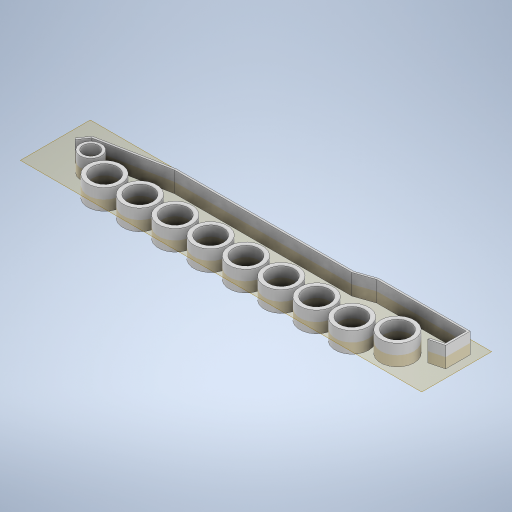
# Autodesk Inventor part: Track_mass_and_inertia
Saved by Autodesk Inventor 2024 (Build 280153000, 153)
## iProperties
Created: 2026-05-25
Part Number: Track_mass_and_inertia
Material: Generic
Document SubType Name: Modeling
Designer: warny
Density: 1 g/cm^3
Appearance: Default
Author: warny
Autodesk Inventor part; units mm, degrees
ref_plane "YZ Plane" through (0, 0, 0) normal (1, 0, 0) x (0, 1, 0)
ref_plane "XY Plane" through (0, 0, 0) normal (0, 0, 1) x (1, 0, 0)
sketch "Sketch1" plane through (0, 0, 0) normal (0, 1, 0) x (-1, 0, 0)
  line L0 (0, -144.8636) -> (0, 84.5516) construction
  line L1 (624.86, 0) -> (-675.46, 0) construction
  line L2 (338.2, 51.778) -> (439.1, -35.05)
  line L3 (439.1, -35.05) -> (421.2, -60.89)
  line L4 (421.2, -60.89) -> (242.5, -95.89)
  line L5 (242.5, -95.89) -> (-209.7, -95.89)
  line L6 (-209.7, -95.89) -> (-256.7, -112.09)
  line L7 (-256.7, -112.09) -> (-489.7, -112.09)
  line L8 (-489.7, -112.09) -> (-489.7, -49.69)
  line L9 (-489.7, -49.69) -> (-453.7, -40.3)
  line L10 (-453.7, -40.3) -> (-431.7, 3.13)
  line L11 (-431.7, 3.13) -> (-349.7, 51.778)
  line L12 (-349.7, 51.778) -> (338.2, 51.778)
  circle A0 centre (393.1, -28.9) radius 27.035
  circle A1 centre (322.2, 6.91) radius 42.8135
  circle A2 centre (232.2, 6.91) radius 42.8135
  circle A3 centre (142.2, 6.91) radius 42.8135
  circle A4 centre (52.2, 6.91) radius 42.8135
  circle A5 centre (-37.8, 6.91) radius 42.8135
  circle A6 centre (-127.8, 6.91) radius 42.8135
  circle A7 centre (-217.8, 6.91) radius 42.8135
  circle A8 centre (-307.8, 6.91) radius 42.8135
  circle A9 centre (-393.7, -22.87) radius 42.8135
  line L13 (435.2892, -31.7707) -> (414.1627, -62.2683)
  line L14 (418.2462, -56.3735) -> (216.4864, -95.89)
  line L15 (-209.7, -90.89) -> (242.015, -90.89)
  line L16 (-489.7, -107.09) -> (-242.1938, -107.09)
  line L17 (-209.7, -90.89) -> (-256.7, -107.09)
  line L18 (-484.7, -107.09) -> (-484.7, -48.3858)
  line L19 (-453.7, -45.3) -> (-453.7, -40.3)
  line L20 (-453.7, -45.3) -> (-484.7, -53.3858)
  point P0 (0, 0)
  dimension "d0" = 51.778
  dimension "d1" = 35.05
  dimension "d2" = 60.89
  dimension "d3" = 95.89
  dimension "d4" = 95.89
  dimension "d5" = 112.09
  dimension "d6" = 112.09
  dimension "d8" = 40.3
  dimension "d9" = 49.69
  dimension "d10" = 3.13
  dimension "d11" = 51.778
  dimension "d12" = 338.2
  dimension "d13" = 439.1
  dimension "d14" = 421.2
  dimension "d15" = 242.5
  dimension "d16" = 489.7
  dimension "d17" = 256.7
  dimension "d18" = 209.7
  dimension "d19" = 489.7
  dimension "d20" = 453.7
  dimension "d21" = 431.7
  dimension "d22" = 349.7
  dimension "d25" = 393.1
  dimension "d26" = 28.9
  dimension "d27" = 54.07
  dimension "d28" = 322.2
  dimension "d29" = 6.91
  dimension "d30" = 85.627
  dimension "d31" = 90
  dimension "d32" = 90
  dimension "d33" = 6.91
  dimension "d34" = 6.91
  dimension "d35" = 90
  dimension "d36" = 6.91
  dimension "d37" = 90
  dimension "d38" = 6.91
  dimension "d39" = 90
  dimension "d40" = 6.91
  dimension "d41" = 90
  dimension "d42" = 6.91
  dimension "d43" = 90
  dimension "d44" = 6.91
  dimension "d45" = 85.627
  dimension "d46" = 85.627
  dimension "d47" = 85.627
  dimension "d48" = 85.627
  dimension "d49" = 85.627
  dimension "d50" = 85.627
  dimension "d51" = 85.627
  dimension "d52" = 393.7
  dimension "d53" = 22.87
  dimension "d54" = 85.627
  dimension "d55" = 5
  dimension "d56" = 5
  dimension "d57" = 5
  dimension "d58" = 209.7
  dimension "d59" = 5
  dimension "d60" = 5
  dimension "d61" = 5
  constraints: 38 end point, 11 point on line, 10 centre point, 10 coincident, 6 parallel, 2 vertical
  measures "d0" distance from line of L2.start L1
  measures "d1" distance from line of L1 L2.end
  measures "d2" distance from line of L1 L3.end
  measures "d3" distance from line of L1 L4.end
  measures "d4" distance from line of L1 L5.end
  measures "d5" distance from line of L1 L6.end
  measures "d6" distance from line of L1 L7.end
  measures "d8" distance from line of L1 L9.end
  measures "d9" distance from line of L1 L8.end
  measures "d10" distance from line of L1 L10.end
  measures "d11" distance from line of L1 L11.end
  measures "d12" distance from line of L2.start L0
  measures "d13" distance from line of L0 L2.end
  measures "d14" distance from line of L0 L3.end
  measures "d15" distance from line of L0 L4.end
  measures "d16" distance from line of L0 L7.end
  measures "d17" distance from line of L0 L6.end
  measures "d18" distance from line of L0 L5.end
  measures "d19" distance from line of L0 L8.end
  measures "d20" distance from line of L0 L9.end
  measures "d21" distance from line of L0 L10.end
  measures "d22" distance from line of L0 L11.end
  measures "d25" distance from line of L0 point (393.1, -28.9)
  measures "d26" distance from line of L1 point (393.1, -28.9)
  measures "d27" diameter of A0
  measures "d28" distance from line of L0 point (322.2, 6.91)
  measures "d29" distance from line of L1 point (322.2, 6.91)
  measures "d30" diameter of A1
  measures "d31" distance of point (232.2, 6.91) point (322.2, 6.91)
  measures "d32" distance of point (232.2, 6.91) point (142.2, 6.91)
  measures "d33" distance from line of L1 point (232.2, 6.91)
  measures "d34" distance from line of L1 point (142.2, 6.91)
  measures "d35" distance of point (142.2, 6.91) point (52.2, 6.91)
  measures "d36" distance from line of L1 point (52.2, 6.91)
  measures "d37" distance of point (52.2, 6.91) point (-37.8, 6.91)
  measures "d38" distance from line of L1 point (-37.8, 6.91)
  measures "d39" distance of point (-127.8, 6.91) point (-37.8, 6.91)
  measures "d40" distance from line of L1 point (-127.8, 6.91)
  measures "d41" distance of point (-127.8, 6.91) point (-217.8, 6.91)
  measures "d42" distance from line of L1 point (-217.8, 6.91)
  measures "d43" distance of point (-217.8, 6.91) point (-307.8, 6.91)
  measures "d44" distance from line of L1 point (-307.8, 6.91)
  measures "d45" diameter of A2
  measures "d46" diameter of A3
  measures "d47" diameter of A4
  measures "d48" diameter of A5
  measures "d49" diameter of A6
  measures "d50" diameter of A7
  measures "d51" diameter of A8
  measures "d52" distance from line of L0 point (-393.7, -22.87)
  measures "d53" distance from line of L1 point (-393.7, -22.87)
  measures "d54" diameter of A9
  measures "d55" distance between parallel lines of L3 L13
  measures "d56" distance between parallel lines of L4 L14
  measures "d57" distance of L15.start L5.end
  measures "d58" distance from line of L0 L15.start
  measures "d59" distance between parallel lines of L16 L7
  measures "d60" distance from line of L18 L8.end
  measures "d61" distance of L9.end L19.start
extrude "Extrusion2" add sketch "Sketch1" along normal mid plane 52 contours L2 L3 L4 L13 | A0 L2 | L2 A0 | L13 L4 L5 L14 | L14 L5 L6 L16 L17 L15 | L16 L6 L7 L8 | A9 L11 | L11 A9 | L16 L8 L9 L18 | L18 L9 L19 L20 | A1 | A2 | A3 | A4 | A5 | A6 | A7 | A8
sketch "Sketch2" plane through (-393.1, 26, -28.9) normal (0, 1, 0) x (1, 0, 0)
  circle A0 centre (0, 0) radius 27.035 projected
  point P0 (393.1, -28.9)
  constraints: 1 coincident
hole "Hole1" at (-393.1, 26, -28.9) direction (0, -1, 0) diameter 40 end through all
sketch "Sketch3" plane through (-322.2, 26, 6.91) normal (0, 1, 0) x (1, 0, 0)
  circle A0 centre (0, 0) radius 42.8135 projected
  circle A1 centre (90, 0) radius 42.8135 projected
  circle A2 centre (180, 0) radius 42.8135 projected
  circle A3 centre (270, 0) radius 42.8135 projected
  circle A4 centre (360, 0) radius 42.8135 projected
  circle A5 centre (450, 0) radius 42.8135 projected
  circle A6 centre (540, 0) radius 42.8135 projected
  circle A7 centre (630, 0) radius 42.8135 projected
  circle A8 centre (715.9, 29.78) radius 42.8135 projected
  point P0 (322.2, 6.91)
  constraints: 9 coincident
hole "Hole2" at (-322.2, 26, 6.91) at (-232.2, 26, 6.91) at (-142.2, 26, 6.91) at (-52.2, 26, 6.91) at (37.8, 26, 6.91) at (127.8, 26, 6.91) at (217.8, 26, 6.91) at (307.8, 26, 6.91) at (393.7, 26, -22.87) direction (0, -1, 0) diameter 65 end through all
body "Solid2"
